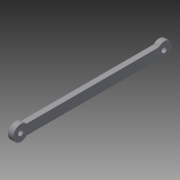
# Autodesk Inventor part: Linkage Arm
Saved by Autodesk Inventor 2015 (Build 190159000, 159)
## iProperties
Created: 2018-03-27
Part Number: Linkage Arm
Material: Generic
Document SubType Name: Modeling
Designer: Administrator
Density: 1 g/cm^3
Appearance: Default
Author: Administrator
Autodesk Inventor part; units mm, degrees
ref_plane "YZ Plane" through (0, 0, 0) normal (1, 0, 0) x (0, 1, 0)
ref_plane "XZ Plane" through (0, 0, 0) normal (0, 1, 0) x (-1, 0, 0)
ref_plane "XY Plane" through (0, 0, 0) normal (0, 0, 1) x (1, 0, 0)
sketch "Sketch1" plane through (0, 0, 0) normal (1, 0, 0) x (0, 1, 0)
  line L0 (10.2056, -9.9502) -> (10.2056, -91.7507)
  arc A0 (10.2056, -9.9502) -> (3.8556, -9.9502) centre (7.0306, -6.4004) ccw
  arc A1 (3.8556, -91.7507) -> (10.2056, -91.7507) centre (7.0306, -95.3004) ccw
  line L1 (3.8556, -9.9502) -> (3.8556, -91.7507)
  point P0 (0, 0)
  dimension "d1" = 88.9
  dimension "d2" = 9.525
  dimension "d5" = 6.35
  dimension "d6" = 9.525
  dimension "d7" = 0
  dimension "d8" = 3.175
  constraints: 4 end point, 4 point on circle, 2 centre point, 2 vertical
  measures "d1" distance of A1.centre A0.centre
  measures "d2" diameter of A0
  measures "d5" distance between parallel lines of L0 L1
  measures "d6" diameter of A1
  measures "d7" horizontal distance of A1.centre A0.centre
  measures "d8" distance from line of L1 A0.centre
extrude "Extrusion1" add sketch "Sketch1" along normal blind 3.175
sketch "Sketch2" plane through (3.175, 0, 0) normal (1, 0, 0) x (0, 0, -1)
  arc A0 (9.9502, 10.2056) -> (9.9502, 3.8556) centre (6.4004, 7.0306) ccw projected
  arc A1 (91.7507, 3.8556) -> (91.7507, 10.2056) centre (95.3004, 7.0306) ccw projected
  point P0 (0, 0)
  constraints: 2 coincident
hole "Hole1" at (3.175, 7.0306, -6.4004) at (3.175, 7.0306, -95.3004) direction (-1, 0, 0) diameter 3.2512 depth 25.4 tip angle 118
body "Solid1"
